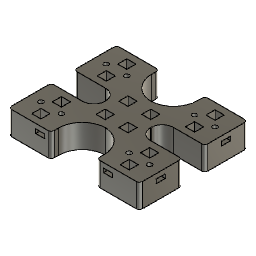
Axis Body (Autodesk Fusion 360 design; units mm, degrees)
Autodesk Fusion 360 part; units mm, degrees
sketch "Sketch1" plane through (0, 0, 0) normal (0, 0, 1) x (1, 0, 0)
  line L0 (14.5, 14.5) -> (-14.5, 14.5)
  line L1 (-14.5, 14.5) -> (-14.5, -14.5)
  line L2 (-14.5, -14.5) -> (-0.5, -14.5)
  line L3 (14.5, -14.5) -> (14.5, 14.5)
  line L4 (-13.5, 13.5) -> (-13.5, 1) construction
  line L5 (-13.5, -1) -> (-13.5, -13.5) construction
  line L6 (-1, -13.5) -> (-1, -1) construction
  line L7 (-1, 1) -> (-1, 13.5) construction
  line L8 (13.5, 1) -> (1, 1) construction
  line L9 (-1, 1) -> (-13.5, 1) construction
  line L10 (1, -13.5) -> (1, -1) construction
  line L11 (1, 1) -> (1, 13.5) construction
  line L12 (14.5, -1) -> (1, -1) construction
  line L13 (-1, -1) -> (-13.5, -1) construction
  line L14 (-13.5, -13.5) -> (-1, -13.5) construction
  line L15 (1, -13.5) -> (13.5, -13.5) construction
  line L16 (13.5, -13.5) -> (13.5, -1) construction
  line L17 (13.5, 1) -> (13.5, 13.5) construction
  line L18 (13.5, 13.5) -> (1, 13.5) construction
  line L19 (-1, 13.5) -> (-13.5, 13.5) construction
  circle A0 centre (7.25, 7.25) radius 6.25 construction
  circle A1 centre (7.25, -7.25) radius 6.25 construction
  circle A2 centre (-7.25, -7.25) radius 6.25 construction
  circle A3 centre (-7.25, 7.25) radius 6.25 construction
  circle A4 centre (7.25, 7.25) radius 1.5
  circle A5 centre (-7.25, 7.25) radius 1.5
  circle A6 centre (-7.25, -7.25) radius 1.5
  circle A7 centre (7.25, -7.25) radius 1.5
  line L20 (7.25, -7.25) -> (19.503, -7.25) construction
  line L21 (14.5, -7.25) -> (41.5, -7.25)
  line L22 (41.5, -7.25) -> (41.5, -34.25)
  line L23 (41.5, -34.25) -> (14.5, -34.25)
  line L24 (14.5, -34.25) -> (14.5, -29.5)
  arc A8 (14.5, -29.5) -> (-0.5, -14.5) centre (-0.5, -29.5) ccw
  line L25 (0, 14.5) -> (0, -40.878) construction
  line L26 (-14.5, -7.25) -> (-41.5, -7.25)
  line L27 (-41.5, -7.25) -> (-41.5, -34.25)
  line L28 (-41.5, -34.25) -> (-14.5, -34.25)
  arc A9 (0.5, -14.5) -> (-14.5, -29.5) centre (0.5, -29.5) ccw
  line L29 (-14.5, -34.25) -> (-14.5, -29.5)
  line L30 (-14.5, 0) -> (32.632, 0) construction
  arc A10 (-0.5, 14.5) -> (14.5, 29.5) centre (-0.5, 29.5) ccw
  line L31 (14.5, 34.25) -> (14.5, 29.5)
  line L32 (41.5, 34.25) -> (14.5, 34.25)
  line L33 (41.5, 7.25) -> (41.5, 34.25)
  line L34 (14.5, 7.25) -> (41.5, 7.25)
  arc A11 (-14.5, 29.5) -> (0.5, 14.5) centre (0.5, 29.5) ccw
  line L35 (-14.5, 34.25) -> (-14.5, 29.5)
  line L36 (-41.5, 34.25) -> (-14.5, 34.25)
  line L37 (-41.5, 7.25) -> (-41.5, 34.25)
  line L38 (-14.5, 7.25) -> (-41.5, 7.25)
  line L39 (28, -34.25) -> (28, -7.25) construction
  line L40 (28, -34.25) -> (28, -27.25) construction
  point P0 (28, -14.25)
  point P1 (28, -27.25)
  point P2 (-28, -14.25)
  point P3 (-28, -27.25)
  point P4 (-28, 14.25)
  point P5 (-28, 27.25)
  point P6 (28, 27.25)
  point P7 (28, 14.25)
  dimension "d1" = 29
  dimension "d2" = 29
  dimension "d13" = 3
  dimension "d14" = 3
  dimension "d15" = 3
  dimension "d16" = 3
  dimension "d17" = 27
  dimension "d18" = 27
  dimension "d19" = 15
  dimension "d22" = 7
  dimension "d23" = 7
  constraint perpendicular L0 L1
  constraint parallel L1 L4
  constraint coincident L4.end L8
  constraint coincident L5.start L12
  constraint collinear L4 L5
  constraint coincident L6.end L12
  constraint coincident L7.start L8
  constraint collinear L6 L7
  constraint coincident L8.end L10
  constraint collinear L8 L9
  constraint collinear L10 L11
  constraint collinear L12 L13
  constraint parallel L2 L14
  constraint collinear L14 L15
  constraint parallel L3 L16
  constraint coincident L12 L16.end
  constraint collinear L16 L17
  constraint parallel L0 L18
  constraint collinear L18 L19
  constraint tangent L18 A0
  constraint tangent L12 A1
  constraint tangent L14 A2
  constraint tangent L19 A3
  constraint concentric A0 A4
  constraint concentric A3 A5
  constraint concentric A2 A6
  constraint concentric A1 A7
  constraint coincident A1.centre A7.centre
  constraint perpendicular L3 L20
  constraint horizontal L21
  constraint vertical L22
  constraint horizontal L23
  constraint vertical L24
  constraint coincident L20 L21.start
  constraint coincident L3 L21.start
  constraint coincident L3.start L2
  constraint coincident L21.start L24
  constraint tangent L2 A8
  constraint tangent L24 A8
  constraint midpoint L0 L25.start
  constraint perpendicular L15 L25
  constraint symmetric L21.start L25 L26.start
  constraint symmetric L21.end L25 L26.end
  constraint symmetric L22.end L25 L27.end
  constraint symmetric L23.end L25 L28.end
  constraint symmetric L2.end L25 A9.start
  constraint symmetric L24.end L25 A9.end
  constraint symmetric A8 L25 A9
  constraint midpoint L1 L30.start
  constraint perpendicular L1 L30
  constraint symmetric L21.start L30 L34.start
  constraint symmetric L21.end L30 L33.start
  constraint symmetric L22.end L30 L32.start
  constraint symmetric L23.end L30 L31.start
  constraint symmetric L2.end L30 A10.start
  constraint symmetric L24.end L30 A10.end
  constraint symmetric A8 L30 A10
  constraint symmetric L26.start L30 L38.start
  constraint symmetric L26.end L30 L37.start
  constraint symmetric L27.end L30 L36.start
  constraint symmetric L28.end L30 L35.start
  constraint symmetric A9.end L30 A11.start
  constraint symmetric A9.start L30 A11.end
  constraint symmetric A9 L30 A11
  constraint midpoint L23 L39.start
  constraint midpoint L21 L39.end
  constraint perpendicular L23 L40
  constraint coincident P1 L40.end
  constraint symmetric L25 P0 P2
  constraint symmetric L25 P1 P3
  constraint symmetric L30 P0 P7
  constraint symmetric L30 P1 P6
  constraint symmetric L30 P2 P4
  constraint symmetric L30 P3 P5
  measures "d1" distance of L1.end L3.start
  measures "d2" distance of L0.end L1.end
  measures "d13" diameter of A4
  measures "d14" diameter of A5
  measures "d15" diameter of A6
  measures "d16" diameter of A7
  measures "d17" distance of L21.start L21.end
  measures "d18" distance of L21.start L23.end
  measures "d19" radius of A8
  measures "d22" distance of L39.end P0
  measures "d23" distance of L39.start P1
  measures "d89" distance of L30.start
  measures "d90" distance of L30.start
extrude "Extrude2" add sketch "Sketch1" along normal blind 15 contours L0 L1 L2 L3 L21 L22 L23 L24 A8 | L0 L3 A10 L31 L32 L33 L34 A11 | L0 L1 A10 A11 L35 L36 L37 L38 | L1 L2 A8 L26 L27 L28 A9 L29 makes body 1
sketch "Sketch2" plane through (0, 0, 15) normal (0, 0, 1) x (-1, 0, 0)
  circle A0 centre (7.25, 7.25) radius 1.5
  circle A1 centre (7.25, -7.25) radius 1.5
  circle A2 centre (-7.25, 7.25) radius 1.5
  circle A3 centre (-7.25, -7.25) radius 1.5
  line L0 (-14.5, 7.25) -> (-14.5, -7.25)
  line L1 (-14.5, -7.25) -> (-41.5, -7.25)
  line L2 (-41.5, -7.25) -> (-41.5, -34.25)
  line L3 (-41.5, -34.25) -> (-14.5, -34.25)
  line L4 (-14.5, -34.25) -> (-14.5, -29.5)
  arc A4 (0, -14.5083) -> (-14.5, -29.5) centre (0.5, -29.5) ccw
  arc A5 (0, -14.5083) -> (-0.5, -14.5) centre (-0.5, -29.5) ccw
  line L5 (-0.5, -14.5) -> (0.5, -14.5)
  arc A6 (0.5, -14.5) -> (0, -14.5083) centre (0.5, -29.5) ccw
  arc A7 (14.5, -29.5) -> (0, -14.5083) centre (-0.5, -29.5) ccw
  line L6 (14.5, -29.5) -> (14.5, -34.25)
  line L7 (14.5, -34.25) -> (41.5, -34.25)
  line L8 (41.5, -34.25) -> (41.5, -7.25)
  line L9 (41.5, -7.25) -> (14.5, -7.25)
  line L10 (14.5, -7.25) -> (14.5, 7.25)
  line L11 (14.5, 7.25) -> (41.5, 7.25)
  line L12 (41.5, 7.25) -> (41.5, 34.25)
  line L13 (41.5, 34.25) -> (14.5, 34.25)
  line L14 (14.5, 34.25) -> (14.5, 29.5)
  arc A8 (0, 14.5083) -> (14.5, 29.5) centre (-0.5, 29.5) ccw
  arc A9 (-14.5, 29.5) -> (0, 14.5083) centre (0.5, 29.5) ccw
  line L15 (-14.5, 29.5) -> (-14.5, 34.25)
  line L16 (-14.5, 34.25) -> (-41.5, 34.25)
  line L17 (-41.5, 34.25) -> (-41.5, 7.25)
  line L18 (-41.5, 7.25) -> (-14.5, 7.25)
  circle A10 centre (-28, 27.25) radius 1.5
  circle A11 centre (-28, 14.25) radius 1.5
  circle A12 centre (-28, -14.25) radius 1.5
  circle A13 centre (-28, -27.25) radius 1.5
  circle A14 centre (28, -27.25) radius 1.5
  circle A15 centre (28, -14.25) radius 1.5
  circle A16 centre (28, 14.25) radius 1.5
  circle A17 centre (28, 27.25) radius 1.5
  point P0 (-28, 27.25)
  point P1 (-28, 14.25)
  point P2 (-28, -14.25)
  point P3 (-28, -27.25)
  point P4 (28, -27.25)
  point P5 (28, -14.25)
  point P6 (28, 14.25)
  point P7 (28, 27.25)
  dimension "d24" = 3
  dimension "d25" = 3
  dimension "d26" = 3
  dimension "d27" = 3
  dimension "d28" = 3
  dimension "d29" = 3
  dimension "d30" = 3
  dimension "d31" = 3
  constraint coincident P0 A10.centre
  constraint coincident P1 A11.centre
  constraint coincident P2 A12.centre
  constraint coincident P3 A13.centre
  constraint coincident P4 A14.centre
  constraint coincident P5 A15.centre
  constraint coincident P6 A16.centre
  constraint coincident P7 A17.centre
  measures "d24" diameter of A10
  measures "d25" diameter of A11
  measures "d26" diameter of A12
  measures "d27" diameter of A13
  measures "d28" diameter of A14
  measures "d29" diameter of A15
  measures "d30" diameter of A16
  measures "d31" diameter of A17
extrude "Extrude3" cut sketch "Sketch2" against normal blind 15 contours A10 | A11 | A12 | A13 | A14 | A15 | A16 | A17 bodies 1
sketch "Sketch3" plane through (0, 0, 15) normal (0, 0, 1) x (-1, 0, 0)
  circle A0 centre (-28, 27.25) radius 1.5
  circle A1 centre (28, -14.25) radius 1.5
  circle A2 centre (28, 14.25) radius 1.5
  circle A3 centre (-28, -27.25) radius 1.5
  circle A4 centre (-28, 14.25) radius 1.5
  circle A5 centre (28, -27.25) radius 1.5
  circle A6 centre (28, 27.25) radius 1.5
  circle A7 centre (-28, -14.25) radius 1.5
  circle A8 centre (7.25, 7.25) radius 1.5
  circle A9 centre (7.25, -7.25) radius 1.5
  circle A10 centre (-7.25, 7.25) radius 1.5
  circle A11 centre (-7.25, -7.25) radius 1.5
  line L0 (-14.5, 7.25) -> (-14.5, -7.25)
  line L1 (-14.5, -7.25) -> (-41.5, -7.25)
  line L2 (-41.5, -7.25) -> (-41.5, -34.25)
  line L3 (-41.5, -34.25) -> (-14.5, -34.25)
  line L4 (-14.5, -34.25) -> (-14.5, -29.5)
  arc A12 (0, -14.5083) -> (-14.5, -29.5) centre (0.5, -29.5) ccw
  arc A13 (0, -14.5083) -> (-0.5, -14.5) centre (-0.5, -29.5) ccw
  line L5 (-0.5, -14.5) -> (0.5, -14.5)
  arc A14 (0.5, -14.5) -> (0, -14.5083) centre (0.5, -29.5) ccw
  arc A15 (14.5, -29.5) -> (0, -14.5083) centre (-0.5, -29.5) ccw
  line L6 (14.5, -29.5) -> (14.5, -34.25)
  line L7 (14.5, -34.25) -> (41.5, -34.25)
  line L8 (41.5, -34.25) -> (41.5, -7.25)
  line L9 (41.5, -7.25) -> (14.5, -7.25)
  line L10 (14.5, -7.25) -> (14.5, 7.25)
  line L11 (14.5, 7.25) -> (41.5, 7.25)
  line L12 (41.5, 7.25) -> (41.5, 34.25)
  line L13 (41.5, 34.25) -> (14.5, 34.25)
  line L14 (14.5, 34.25) -> (14.5, 29.5)
  arc A16 (0, 14.5083) -> (14.5, 29.5) centre (-0.5, 29.5) ccw
  arc A17 (-14.5, 29.5) -> (0, 14.5083) centre (0.5, 29.5) ccw
  line L15 (-14.5, 29.5) -> (-14.5, 34.25)
  line L16 (-14.5, 34.25) -> (-41.5, 34.25)
  line L17 (-41.5, 34.25) -> (-41.5, 7.25)
  line L18 (-41.5, 7.25) -> (-14.5, 7.25)
  line L19 (-30.875, -24.375) -> (-25.125, -24.375)
  line L20 (-25.125, -24.375) -> (-25.125, -30.125)
  line L21 (-25.125, -30.125) -> (-30.875, -30.125)
  line L22 (-30.875, -30.125) -> (-30.875, -24.375)
  line L23 (-30.875, -24.375) -> (-25.125, -30.125) construction
  line L24 (-25.125, -24.375) -> (-30.875, -30.125) construction
  line L25 (-30.875, -11.375) -> (-25.125, -11.375)
  line L26 (-25.125, -11.375) -> (-25.125, -17.125)
  line L27 (-25.125, -17.125) -> (-30.875, -17.125)
  line L28 (-30.875, -17.125) -> (-30.875, -11.375)
  line L29 (-30.875, -11.375) -> (-25.125, -17.125) construction
  line L30 (-25.125, -11.375) -> (-30.875, -17.125) construction
  line L31 (-10.125, -4.375) -> (-4.375, -4.375)
  line L32 (-4.375, -4.375) -> (-4.375, -10.125)
  line L33 (-4.375, -10.125) -> (-10.125, -10.125)
  line L34 (-10.125, -10.125) -> (-10.125, -4.375)
  line L35 (-10.125, -4.375) -> (-4.375, -10.125) construction
  line L36 (-4.375, -4.375) -> (-10.125, -10.125) construction
  line L37 (4.375, -4.375) -> (10.125, -4.375)
  line L38 (10.125, -4.375) -> (10.125, -10.125)
  line L39 (10.125, -10.125) -> (4.375, -10.125)
  line L40 (4.375, -10.125) -> (4.375, -4.375)
  line L41 (4.375, -4.375) -> (10.125, -10.125) construction
  line L42 (10.125, -4.375) -> (4.375, -10.125) construction
  line L43 (25.125, -11.375) -> (30.875, -11.375)
  line L44 (30.875, -11.375) -> (30.875, -17.125)
  line L45 (30.875, -17.125) -> (25.125, -17.125)
  line L46 (25.125, -17.125) -> (25.125, -11.375)
  line L47 (25.125, -11.375) -> (30.875, -17.125) construction
  line L48 (30.875, -11.375) -> (25.125, -17.125) construction
  line L49 (25.125, -24.375) -> (30.875, -24.375)
  line L50 (30.875, -24.375) -> (30.875, -30.125)
  line L51 (30.875, -30.125) -> (25.125, -30.125)
  line L52 (25.125, -30.125) -> (25.125, -24.375)
  line L53 (25.125, -24.375) -> (30.875, -30.125) construction
  line L54 (30.875, -24.375) -> (25.125, -30.125) construction
  line L55 (-10.125, 10.125) -> (-4.375, 10.125)
  line L56 (-4.375, 10.125) -> (-4.375, 4.375)
  line L57 (-4.375, 4.375) -> (-10.125, 4.375)
  line L58 (-10.125, 4.375) -> (-10.125, 10.125)
  line L59 (-10.125, 10.125) -> (-4.375, 4.375) construction
  line L60 (-4.375, 10.125) -> (-10.125, 4.375) construction
  line L61 (4.375, 10.125) -> (10.125, 10.125)
  line L62 (10.125, 10.125) -> (10.125, 4.375)
  line L63 (10.125, 4.375) -> (4.375, 4.375)
  line L64 (4.375, 4.375) -> (4.375, 10.125)
  line L65 (4.375, 10.125) -> (10.125, 4.375) construction
  line L66 (10.125, 10.125) -> (4.375, 4.375) construction
  line L67 (-30.875, 17.125) -> (-25.125, 17.125)
  line L68 (-25.125, 17.125) -> (-25.125, 11.375)
  line L69 (-25.125, 11.375) -> (-30.875, 11.375)
  line L70 (-30.875, 11.375) -> (-30.875, 17.125)
  line L71 (-30.875, 17.125) -> (-25.125, 11.375) construction
  line L72 (-25.125, 17.125) -> (-30.875, 11.375) construction
  line L73 (-30.875, 30.125) -> (-25.125, 30.125)
  line L74 (-25.125, 30.125) -> (-25.125, 24.375)
  line L75 (-25.125, 24.375) -> (-30.875, 24.375)
  line L76 (-30.875, 24.375) -> (-30.875, 30.125)
  line L77 (-30.875, 30.125) -> (-25.125, 24.375) construction
  line L78 (-25.125, 30.125) -> (-30.875, 24.375) construction
  line L79 (25.125, 17.125) -> (30.875, 17.125)
  line L80 (30.875, 17.125) -> (30.875, 11.375)
  line L81 (30.875, 11.375) -> (25.125, 11.375)
  line L82 (25.125, 11.375) -> (25.125, 17.125)
  line L83 (25.125, 17.125) -> (30.875, 11.375) construction
  line L84 (30.875, 17.125) -> (25.125, 11.375) construction
  line L85 (25.125, 30.125) -> (30.875, 30.125)
  line L86 (30.875, 30.125) -> (30.875, 24.375)
  line L87 (30.875, 24.375) -> (25.125, 24.375)
  line L88 (25.125, 24.375) -> (25.125, 30.125)
  line L89 (25.125, 30.125) -> (30.875, 24.375) construction
  line L90 (30.875, 30.125) -> (25.125, 24.375) construction
  point P0 (-28, -27.25)
  point P1 (-28, -14.25)
  point P2 (-7.25, -7.25)
  point P3 (7.25, -7.25)
  point P4 (28, -14.25)
  point P5 (28, -27.25)
  point P6 (-7.25, 7.25)
  point P7 (7.25, 7.25)
  point P8 (-28, 14.25)
  point P9 (-28, 27.25)
  point P10 (28, 14.25)
  point P11 (28, 27.25)
  dimension "d34" = 5.75
  dimension "d35" = 5.75
  dimension "d36" = 5.75
  dimension "d37" = 5.75
  dimension "d38" = 5.75
  dimension "d39" = 5.75
  dimension "d40" = 5.75
  dimension "d41" = 5.75
  dimension "d42" = 5.75
  dimension "d43" = 5.75
  dimension "d44" = 5.75
  dimension "d45" = 5.75
  dimension "d46" = 5.75
  dimension "d47" = 5.75
  dimension "d48" = 5.75
  dimension "d49" = 5.75
  dimension "d50" = 5.75
  dimension "d51" = 5.75
  dimension "d52" = 5.75
  dimension "d53" = 5.75
  dimension "d54" = 5.75
  dimension "d55" = 5.75
  dimension "d56" = 5.75
  dimension "d57" = 5.75
  constraint horizontal L19
  constraint perpendicular L19 L20
  constraint parallel L19 L21
  constraint parallel L20 L22
  constraint coincident L23 P0
  constraint coincident L24 P0
  constraint coincident P0 A3.centre
  constraint horizontal L25
  constraint perpendicular L25 L26
  constraint parallel L25 L27
  constraint parallel L26 L28
  constraint coincident L29 P1
  constraint coincident L30 P1
  constraint coincident P1 A7.centre
  constraint horizontal L31
  constraint perpendicular L31 L32
  constraint parallel L31 L33
  constraint parallel L32 L34
  constraint coincident L35 P2
  constraint coincident L36 P2
  constraint coincident P2 A11.centre
  constraint horizontal L37
  constraint perpendicular L37 L38
  constraint parallel L37 L39
  constraint parallel L38 L40
  constraint coincident L41 P3
  constraint coincident L42 P3
  constraint coincident P3 A9.centre
  constraint horizontal L43
  constraint perpendicular L43 L44
  constraint parallel L43 L45
  constraint parallel L44 L46
  constraint coincident L47 P4
  constraint coincident L48 P4
  constraint coincident P4 A1.centre
  constraint horizontal L49
  constraint perpendicular L49 L50
  constraint parallel L49 L51
  constraint parallel L50 L52
  constraint coincident L53 P5
  constraint coincident L54 P5
  constraint coincident P5 A5.centre
  constraint horizontal L55
  constraint perpendicular L55 L56
  constraint parallel L55 L57
  constraint parallel L56 L58
  constraint coincident L59 P6
  constraint coincident L60 P6
  constraint coincident P6 A10.centre
  constraint horizontal L61
  constraint perpendicular L61 L62
  constraint parallel L61 L63
  constraint parallel L62 L64
  constraint coincident L65 P7
  constraint coincident L66 P7
  constraint coincident P7 A8.centre
  constraint horizontal L67
  constraint perpendicular L67 L68
  constraint parallel L67 L69
  constraint parallel L68 L70
  constraint coincident L71 P8
  constraint coincident L72 P8
  constraint coincident P8 A4.centre
  constraint horizontal L73
  constraint perpendicular L73 L74
  constraint parallel L73 L75
  constraint parallel L74 L76
  constraint coincident L77 P9
  constraint coincident L78 P9
  constraint coincident P9 A0.centre
  constraint horizontal L79
  constraint perpendicular L79 L80
  constraint parallel L79 L81
  constraint parallel L80 L82
  constraint coincident L83 P10
  constraint coincident L84 P10
  constraint coincident P10 A2.centre
  constraint horizontal L85
  constraint perpendicular L85 L86
  constraint parallel L85 L87
  constraint parallel L86 L88
  constraint coincident L89 P11
  constraint coincident L90 P11
  constraint coincident P11 A6.centre
  measures "d34" distance of L20.end L21.end
  measures "d35" distance of L19.end L20.end
  measures "d36" distance of L26.end L27.end
  measures "d37" distance of L25.end L26.end
  measures "d38" distance of L32.end L33.end
  measures "d39" distance of L31.end L32.end
  measures "d40" distance of L38.end L39.end
  measures "d41" distance of L37.end L38.end
  measures "d42" distance of L44.end L45.end
  measures "d43" distance of L43.end L44.end
  measures "d44" distance of L50.end L51.end
  measures "d45" distance of L49.end L50.end
  measures "d46" distance of L56.end L57.end
  measures "d47" distance of L55.end L56.end
  measures "d48" distance of L62.end L63.end
  measures "d49" distance of L61.end L62.end
  measures "d50" distance of L68.end L69.end
  measures "d51" distance of L67.end L68.end
  measures "d52" distance of L74.end L75.end
  measures "d53" distance of L73.end L74.end
  measures "d54" distance of L80.end L81.end
  measures "d55" distance of L79.end L80.end
  measures "d56" distance of L86.end L87.end
  measures "d57" distance of L85.end L86.end
extrude "Extrude4" cut sketch "Sketch3" against normal blind 7.5 contours L19 L20 L21 L22 | L25 L26 L27 L28 | L31 L32 L33 L34 | L37 L38 L39 L40 | L43 L44 L45 L46 | L49 L50 L51 L52 | L55 L56 L57 L58 | L61 L62 L63 L64 | L67 L68 L69 L70 | L73 L74 L75 L76 | L79 L80 L81 L82 | L85 L86 L87 L88 bodies 1
sketch "Sketch4" plane through (0, 0, 15) normal (0, 0, 1) x (-1, 0, 0)
  line L0 (-25.125, -24.375) -> (-25.125, -30.125)
  line L1 (-25.125, -30.125) -> (-30.875, -30.125)
  line L2 (-30.875, -30.125) -> (-30.875, -24.375)
  line L3 (-30.875, -24.375) -> (-25.125, -24.375)
  line L4 (10.125, 10.125) -> (10.125, 4.375)
  line L5 (10.125, 4.375) -> (4.375, 4.375)
  line L6 (4.375, 4.375) -> (4.375, 10.125)
  line L7 (4.375, 10.125) -> (10.125, 10.125)
  line L8 (30.875, 17.125) -> (30.875, 11.375)
  line L9 (30.875, 11.375) -> (25.125, 11.375)
  line L10 (25.125, 11.375) -> (25.125, 17.125)
  line L11 (25.125, 17.125) -> (30.875, 17.125)
  line L12 (30.875, -11.375) -> (30.875, -17.125)
  line L13 (30.875, -17.125) -> (25.125, -17.125)
  line L14 (25.125, -17.125) -> (25.125, -11.375)
  line L15 (25.125, -11.375) -> (30.875, -11.375)
  line L16 (-4.375, 10.125) -> (-4.375, 4.375)
  line L17 (-4.375, 4.375) -> (-10.125, 4.375)
  line L18 (-10.125, 4.375) -> (-10.125, 10.125)
  line L19 (-10.125, 10.125) -> (-4.375, 10.125)
  line L20 (-25.125, 17.125) -> (-25.125, 11.375)
  line L21 (-25.125, 11.375) -> (-30.875, 11.375)
  line L22 (-30.875, 11.375) -> (-30.875, 17.125)
  line L23 (-30.875, 17.125) -> (-25.125, 17.125)
  line L24 (-25.125, -11.375) -> (-25.125, -17.125)
  line L25 (-25.125, -17.125) -> (-30.875, -17.125)
  line L26 (-30.875, -17.125) -> (-30.875, -11.375)
  line L27 (-30.875, -11.375) -> (-25.125, -11.375)
  line L28 (10.125, -4.375) -> (10.125, -10.125)
  line L29 (10.125, -10.125) -> (4.375, -10.125)
  line L30 (4.375, -10.125) -> (4.375, -4.375)
  line L31 (4.375, -4.375) -> (10.125, -4.375)
  line L32 (30.875, 30.125) -> (30.875, 24.375)
  line L33 (30.875, 24.375) -> (25.125, 24.375)
  line L34 (25.125, 24.375) -> (25.125, 30.125)
  line L35 (25.125, 30.125) -> (30.875, 30.125)
  line L36 (30.875, -24.375) -> (30.875, -30.125)
  line L37 (30.875, -30.125) -> (25.125, -30.125)
  line L38 (25.125, -30.125) -> (25.125, -24.375)
  line L39 (25.125, -24.375) -> (30.875, -24.375)
  line L40 (-4.375, -4.375) -> (-4.375, -10.125)
  line L41 (-4.375, -10.125) -> (-10.125, -10.125)
  line L42 (-10.125, -10.125) -> (-10.125, -4.375)
  line L43 (-10.125, -4.375) -> (-4.375, -4.375)
  line L44 (-25.125, 30.125) -> (-25.125, 24.375)
  line L45 (-25.125, 24.375) -> (-30.875, 24.375)
  line L46 (-30.875, 24.375) -> (-30.875, 30.125)
  line L47 (-30.875, 30.125) -> (-25.125, 30.125)
  line L48 (-14.5, 7.25) -> (-14.5, -7.25)
  line L49 (-14.5, -7.25) -> (-41.5, -7.25)
  line L50 (-41.5, -7.25) -> (-41.5, -34.25)
  line L51 (-41.5, -34.25) -> (-14.5, -34.25)
  line L52 (-14.5, -34.25) -> (-14.5, -29.5)
  arc A0 (0, -14.5083) -> (-14.5, -29.5) centre (0.5, -29.5) ccw
  arc A1 (0, -14.5083) -> (-0.5, -14.5) centre (-0.5, -29.5) ccw
  line L53 (-0.5, -14.5) -> (0.5, -14.5)
  arc A2 (0.5, -14.5) -> (0, -14.5083) centre (0.5, -29.5) ccw
  arc A3 (14.5, -29.5) -> (0, -14.5083) centre (-0.5, -29.5) ccw
  line L54 (14.5, -29.5) -> (14.5, -34.25)
  line L55 (14.5, -34.25) -> (41.5, -34.25)
  line L56 (41.5, -34.25) -> (41.5, -7.25)
  line L57 (41.5, -7.25) -> (14.5, -7.25)
  line L58 (14.5, -7.25) -> (14.5, 7.25)
  line L59 (14.5, 7.25) -> (41.5, 7.25)
  line L60 (41.5, 7.25) -> (41.5, 34.25)
  line L61 (41.5, 34.25) -> (14.5, 34.25)
  line L62 (14.5, 34.25) -> (14.5, 29.5)
  arc A4 (0, 14.5083) -> (14.5, 29.5) centre (-0.5, 29.5) ccw
  arc A5 (-14.5, 29.5) -> (0, 14.5083) centre (0.5, 29.5) ccw
  line L63 (-14.5, 29.5) -> (-14.5, 34.25)
  line L64 (-14.5, 34.25) -> (-41.5, 34.25)
  line L65 (-41.5, 34.25) -> (-41.5, 7.25)
  line L66 (-41.5, 7.25) -> (-14.5, 7.25)
  line L67 (-41.5, -20.75) -> (-14.0261, -20.75) construction
  line L68 (-41.5, -20.75) -> (-34.5, -20.75) construction
  line L69 (-34.5, -20.75) -> (-21.5, -20.75) construction
  circle A6 centre (-34.5, -20.75) radius 1.5
  circle A7 centre (-21.5, -20.75) radius 1.5
  dimension "d60" = 7
  dimension "d61" = 13
  dimension "d62" = 3
  dimension "d63" = 3
  constraint midpoint L50 L67.start
  constraint perpendicular L50 L67
  constraint perpendicular L50 L68
  constraint parallel L67 L69
  constraint coincident L68.end L69.start
  constraint coincident L69.end A7.centre
  measures "d60" distance of L67.start L68.end
  measures "d61" distance of L68.end L69.end
  measures "d62" diameter of A6
  measures "d63" diameter of A7
extrude "Extrude5" cut sketch "Sketch4" against normal blind 15 contours A6 | A7 bodies 1
mirror "Mirror1" about plane through (0, 0, 0) normal (0, 1, 0) of "Extrude5"
mirror "Mirror2" about plane through (0, 0, 0) normal (1, 0, 0) of "Extrude5", "Mirror1"
sketch "Sketch7" plane through (41.5, 0, 0) normal (1, 0, 0) x (0, 1, 0)
  line L0 (7.25, 0) -> (34.25, 0)
  line L1 (34.25, 0) -> (34.25, 15)
  line L2 (34.25, 15) -> (7.25, 15)
  line L3 (7.25, 15) -> (7.25, 0)
  line L4 (20.75, 15) -> (20.75, 0) construction
  line L5 (20.75, 15) -> (20.75, 12) construction
  line L6 (20.75, 12) -> (20.75, 10.725) construction
  line L7 (23.625, 12) -> (17.875, 12)
  line L8 (17.875, 12) -> (17.875, 9.45)
  line L9 (17.875, 9.45) -> (23.625, 9.45)
  line L10 (23.625, 9.45) -> (23.625, 12)
  line L11 (23.625, 12) -> (17.875, 9.45) construction
  line L12 (17.875, 12) -> (23.625, 9.45) construction
  point P0 (20.75, 10.725)
  dimension "d83" = 3
  dimension "d84" = 1.275
  dimension "d85" = 5.75
  dimension "d86" = 2.55
  constraint midpoint L2 L4.start
  constraint midpoint L0 L4.end
  constraint perpendicular L2 L5
  constraint parallel L4 L6
  constraint horizontal L7
  constraint perpendicular L7 L8
  constraint parallel L7 L9
  constraint parallel L8 L10
  constraint coincident L11 P0
  constraint coincident L12 P0
  constraint coincident P0 L6.end
  measures "d83" distance of L4.start L5.end
  measures "d84" distance of L5.end P0
  measures "d85" distance of L8.end L9.end
  measures "d86" distance of L7.end L8.end
sketch "Sketch8" plane through (0, 34.25, 0) normal (0, 1, 0) x (-1, 0, 0)
  line L0 (-41.5, 0) -> (-14.5, 0)
  line L1 (-14.5, 0) -> (-14.5, 15)
  line L2 (-14.5, 15) -> (-41.5, 15)
  line L3 (-41.5, 15) -> (-41.5, 0)
  line L4 (-41.5, 15) -> (-41.5, 10.725) construction
  line L5 (-41.5, 10.725) -> (-14.5, 10.725) construction
  line L6 (-14.5, 15) -> (-21.5, 15) construction
  line L7 (-21.5, 15) -> (-21.5, 0) construction
  line L8 (-18.625, 9.45) -> (-24.375, 9.45)
  line L9 (-24.375, 9.45) -> (-24.375, 12)
  line L10 (-24.375, 12) -> (-18.625, 12)
  line L11 (-18.625, 12) -> (-18.625, 9.45)
  line L12 (-18.625, 9.45) -> (-24.375, 12) construction
  line L13 (-24.375, 9.45) -> (-18.625, 12) construction
  point P0 (-21.5, 10.725)
  dimension "d87" = 4.275
  dimension "d88" = 7
  dimension "d89" = 5.75
  dimension "d90" = 2.55
  constraint coincident L2.end L3.start
  constraint perpendicular L2 L4
  constraint coincident L1 L5.end
  constraint perpendicular L1 L5
  constraint coincident L1.end L2.start
  constraint perpendicular L1 L6
  constraint coincident L0 L7.end
  constraint perpendicular L0 L7
  constraint horizontal L8
  constraint perpendicular L8 L9
  constraint parallel L8 L10
  constraint parallel L9 L11
  constraint coincident L12 P0
  constraint coincident L13 P0
  constraint coincident L5 P0
  constraint coincident L7 P0
  measures "d87" distance of L2.end L4.end
  measures "d88" distance of L1.end L6.end
  measures "d89" distance of L9.end L10.end
  measures "d90" distance of L8.end L9.end
extrude "Extrude8" cut sketch "Sketch7" against normal blind 9.9 contours L7 L8 L9 L10 bodies 1
extrude "Extrude9" cut sketch "Sketch8" against normal blind 16.45 contours L8 L9 L10 L11 bodies 1
mirror "Mirror5" about plane through (0, 0, 0) normal (0, 1, 0) of "Extrude8", "Extrude9"
mirror "Mirror6" about plane through (0, 0, 0) normal (1, 0, 0) of "Extrude8", "Extrude9", "Mirror5"
copy_body "Body->Comp1" bodies 1 removing the originals makes body 2 in component "Axis Body"
fillet "Fillet1" radius 7 4 edges at (14.5, 7.25, 7.5) (14.5, -7.25, 7.5) (-14.5, 7.25, 7.5) (-14.5, -7.25, 7.5) on bodies 2 in component "Axis Body"
fillet "Fillet2" radius 2 12 edges at (41.5, 7.25, 7.5) (41.5, -7.25, 7.5) (41.5, -34.25, 7.5) (14.5, -34.25, 7.5) (41.5, 34.25, 7.5) (14.5, 34.25, 7.5) (-14.5, 34.25, 7.5) (-41.5, 34.25, 7.5) (-41.5, 7.25, 7.5) (-41.5, -7.25, 7.5) (-41.5, -34.25, 7.5) (-14.5, -34.25, 7.5) on bodies 2 in component "Axis Body"
sketch "Sketch11" plane through (0, 0, 15) normal (0, 0, 1) x (-1, 0, 0)
  circle A0 centre (21.5, 20.75) radius 1.5
  circle A1 centre (34.5, 20.75) radius 1.5
  circle A2 centre (21.5, -20.75) radius 1.5
  circle A3 centre (34.5, -20.75) radius 1.5
  circle A4 centre (-21.5, 20.75) radius 1.5
  circle A5 centre (-34.5, 20.75) radius 1.5
  circle A6 centre (-21.5, -20.75) radius 1.5
  circle A7 centre (-34.5, -20.75) radius 1.5
  line L0 (-25.125, -24.375) -> (-25.125, -30.125)
  line L1 (-25.125, -30.125) -> (-30.875, -30.125)
  line L2 (-30.875, -30.125) -> (-30.875, -24.375)
  line L3 (-30.875, -24.375) -> (-25.125, -24.375)
  line L4 (10.125, 10.125) -> (10.125, 4.375)
  line L5 (10.125, 4.375) -> (4.375, 4.375)
  line L6 (4.375, 4.375) -> (4.375, 10.125)
  line L7 (4.375, 10.125) -> (10.125, 10.125)
  line L8 (30.875, 17.125) -> (30.875, 11.375)
  line L9 (30.875, 11.375) -> (25.125, 11.375)
  line L10 (25.125, 11.375) -> (25.125, 17.125)
  line L11 (25.125, 17.125) -> (30.875, 17.125)
  line L12 (30.875, -11.375) -> (30.875, -17.125)
  line L13 (30.875, -17.125) -> (25.125, -17.125)
  line L14 (25.125, -17.125) -> (25.125, -11.375)
  line L15 (25.125, -11.375) -> (30.875, -11.375)
  line L16 (-4.375, 10.125) -> (-4.375, 4.375)
  line L17 (-4.375, 4.375) -> (-10.125, 4.375)
  line L18 (-10.125, 4.375) -> (-10.125, 10.125)
  line L19 (-10.125, 10.125) -> (-4.375, 10.125)
  line L20 (-25.125, 17.125) -> (-25.125, 11.375)
  line L21 (-25.125, 11.375) -> (-30.875, 11.375)
  line L22 (-30.875, 11.375) -> (-30.875, 17.125)
  line L23 (-30.875, 17.125) -> (-25.125, 17.125)
  line L24 (-25.125, -11.375) -> (-25.125, -17.125)
  line L25 (-25.125, -17.125) -> (-30.875, -17.125)
  line L26 (-30.875, -17.125) -> (-30.875, -11.375)
  line L27 (-30.875, -11.375) -> (-25.125, -11.375)
  line L28 (10.125, -4.375) -> (10.125, -10.125)
  line L29 (10.125, -10.125) -> (4.375, -10.125)
  line L30 (4.375, -10.125) -> (4.375, -4.375)
  line L31 (4.375, -4.375) -> (10.125, -4.375)
  line L32 (30.875, 30.125) -> (30.875, 24.375)
  line L33 (30.875, 24.375) -> (25.125, 24.375)
  line L34 (25.125, 24.375) -> (25.125, 30.125)
  line L35 (25.125, 30.125) -> (30.875, 30.125)
  line L36 (30.875, -24.375) -> (30.875, -30.125)
  line L37 (30.875, -30.125) -> (25.125, -30.125)
  line L38 (25.125, -30.125) -> (25.125, -24.375)
  line L39 (25.125, -24.375) -> (30.875, -24.375)
  line L40 (-4.375, -4.375) -> (-4.375, -10.125)
  line L41 (-4.375, -10.125) -> (-10.125, -10.125)
  line L42 (-10.125, -10.125) -> (-10.125, -4.375)
  line L43 (-10.125, -4.375) -> (-4.375, -4.375)
  line L44 (-25.125, 30.125) -> (-25.125, 24.375)
  line L45 (-25.125, 24.375) -> (-30.875, 24.375)
  line L46 (-30.875, 24.375) -> (-30.875, 30.125)
  line L47 (-30.875, 30.125) -> (-25.125, 30.125)
  arc A8 (16.5, 34.25) -> (14.5, 32.25) centre (16.5, 32.25) ccw
  line L48 (14.5, 32.25) -> (14.5, 29.5)
  arc A9 (0, 14.5083) -> (14.5, 29.5) centre (-0.5, 29.5) ccw
  arc A10 (-14.5, 29.5) -> (0, 14.5083) centre (0.5, 29.5) ccw
  line L49 (-14.5, 29.5) -> (-14.5, 32.25)
  arc A11 (-14.5, 32.25) -> (-16.5, 34.25) centre (-16.5, 32.25) ccw
  line L50 (-16.5, 34.25) -> (-39.5, 34.25)
  arc A12 (-39.5, 34.25) -> (-41.5, 32.25) centre (-39.5, 32.25) ccw
  line L51 (-41.5, 32.25) -> (-41.5, 9.25)
  arc A13 (-41.5, 9.25) -> (-39.5, 7.25) centre (-39.5, 9.25) ccw
  line L52 (-39.5, 7.25) -> (-21.5, 7.25)
  arc A14 (-14.5, 0.25) -> (-21.5, 7.25) centre (-21.5, 0.25) ccw
  line L53 (-14.5, 0.25) -> (-14.5, -0.25)
  arc A15 (-21.5, -7.25) -> (-14.5, -0.25) centre (-21.5, -0.25) ccw
  line L54 (-21.5, -7.25) -> (-39.5, -7.25)
  arc A16 (-39.5, -7.25) -> (-41.5, -9.25) centre (-39.5, -9.25) ccw
  line L55 (-41.5, -9.25) -> (-41.5, -32.25)
  arc A17 (-41.5, -32.25) -> (-39.5, -34.25) centre (-39.5, -32.25) ccw
  line L56 (-39.5, -34.25) -> (-16.5, -34.25)
  arc A18 (-16.5, -34.25) -> (-14.5, -32.25) centre (-16.5, -32.25) ccw
  line L57 (-14.5, -32.25) -> (-14.5, -29.5)
  arc A19 (0, -14.5083) -> (-14.5, -29.5) centre (0.5, -29.5) ccw
  arc A20 (0, -14.5083) -> (-0.5, -14.5) centre (-0.5, -29.5) ccw
  line L58 (-0.5, -14.5) -> (0.5, -14.5)
  arc A21 (0.5, -14.5) -> (0, -14.5083) centre (0.5, -29.5) ccw
  arc A22 (14.5, -29.5) -> (0, -14.5083) centre (-0.5, -29.5) ccw
  line L59 (14.5, -29.5) -> (14.5, -32.25)
  arc A23 (14.5, -32.25) -> (16.5, -34.25) centre (16.5, -32.25) ccw
  line L60 (16.5, -34.25) -> (39.5, -34.25)
  arc A24 (39.5, -34.25) -> (41.5, -32.25) centre (39.5, -32.25) ccw
  line L61 (41.5, -32.25) -> (41.5, -9.25)
  arc A25 (41.5, -9.25) -> (39.5, -7.25) centre (39.5, -9.25) ccw
  line L62 (39.5, -7.25) -> (21.5, -7.25)
  arc A26 (14.5, -0.25) -> (21.5, -7.25) centre (21.5, -0.25) ccw
  line L63 (14.5, -0.25) -> (14.5, 0.25)
  arc A27 (21.5, 7.25) -> (14.5, 0.25) centre (21.5, 0.25) ccw
  line L64 (21.5, 7.25) -> (39.5, 7.25)
  arc A28 (39.5, 7.25) -> (41.5, 9.25) centre (39.5, 9.25) ccw
  line L65 (41.5, 9.25) -> (41.5, 32.25)
  arc A29 (41.5, 32.25) -> (39.5, 34.25) centre (39.5, 32.25) ccw
  line L66 (39.5, 34.25) -> (16.5, 34.25)
  line L67 (28, 34.25) -> (28, 7.25) construction
  circle A30 centre (28, 27.25) radius 1.5 construction
  line L68 (-28, 34.25) -> (-28, 7.25) construction
  constraint midpoint L66 L67.start
  constraint coincident L64 L67.end
  constraint perpendicular L64 L67
  constraint midpoint L50 L68.start
  constraint coincident L52 L68.end
  constraint perpendicular L52 L68
sketch "Sketch12" plane through (0, -34.25, 0) normal (0, -1, 0) x (1, 0, 0)
  line L0 (16.5, 15) -> (16.5, 0)
  line L1 (16.5, 0) -> (39.5, 0)
  line L2 (39.5, 0) -> (39.5, 15)
  line L3 (39.5, 15) -> (16.5, 15)
  line L4 (24.375, 12) -> (24.375, 9.45)
  line L5 (24.375, 9.45) -> (18.625, 9.45)
  line L6 (18.625, 9.45) -> (18.625, 12)
  line L7 (18.625, 12) -> (24.375, 12)
component "Axis Body" placed x (1, 0, 0) y (0, 1, 0) z (0, 0, 1) at (0, 0, 0)
equation "d87 = 3 mm + 1.275 mm"
